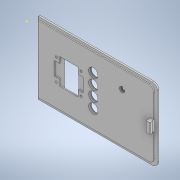
# Autodesk Inventor part: Case top
Saved by Autodesk Inventor 2021 (Build 250183000, 183)
## iProperties
Created: 2020-08-28
Part Number: Case top
Material: Generisch
Document SubType Name: Modeling
Designer: michox
Density: 1 g/cm^3
Appearance: Vorgabe
Author: michox
Autodesk Inventor part; units mm, degrees
ref_plane "YZ Plane" through (0, 0, 0) normal (1, 0, 0) x (0, 1, 0)
ref_plane "XZ Plane" through (0, 0, 0) normal (0, 1, 0) x (-1, 0, 0)
ref_plane "XY Plane" through (0, 0, 0) normal (0, 0, 1) x (1, 0, 0)
sketch "Skizze1" plane through (0, 0, 0) normal (0, 0, 1) x (1, 0, 0)
  line L0 (11.1165, 10) -> (126.7755, 10)
  line L1 (126.7755, 10) -> (126.7755, -60)
  line L2 (126.7755, -60) -> (11.1165, -60)
  line L3 (11.1165, -60) -> (11.1165, 10)
  line L4 (36.6476, -12.5) -> (50.6476, -12.5)
  line L5 (50.6476, -12.5) -> (50.6476, -37.5)
  line L6 (50.6476, -37.5) -> (36.6476, -37.5)
  line L7 (36.6476, -37.5) -> (36.6476, -12.5)
  line L8 (126.7755, -25) -> (11.1165, -25)
  line L9 (126.7755, -36.2282) -> (128.5882, -36.2282)
  line L10 (128.5882, -36.2282) -> (128.5882, -13.7718)
  line L11 (128.5882, -13.7718) -> (126.7755, -13.7718)
  line L12 (126.7755, -13.7718) -> (126.7755, -36.2282)
  circle A0 centre (65.6476, -10) radius 4.5
  circle A1 centre (65.6476, -20) radius 4.5
  circle A2 centre (65.6476, -30) radius 4.5
  circle A3 centre (65.6476, -40) radius 4.5
  circle A4 centre (93.6476, -10) radius 2.5
  point P0 (0, 0)
  dimension "d0" = 115.659
  dimension "d1" = 70
  dimension "d2" = 25
  dimension "d3" = 14
  dimension "d65" = 9
  dimension "d66" = 9
  dimension "d67" = 9
  dimension "d68" = 9
  dimension "d69" = 10
  dimension "d70" = 10
  dimension "d71" = 10
  dimension "d73" = 10
  dimension "d74" = 15
  dimension "d75" = 25.5312
  dimension "d76" = 22.5
  dimension "d77" = 5
  dimension "d79" = 28
  constraints: 26 end point, 6 parallel, 5 centre point, 3 horizontal, 3 perpendicular, 2 midpoint, 1 horizontal alignment, 1 point on line, 1 vertical alignment, 2 other
  measures "d0" distance of L1.end L2.end
  measures "d1" distance of L0.end L1.end
  measures "d2" distance of L4.end L5.end
  measures "d3" distance of L4.start L4.end
  measures "d65" diameter of A0
  measures "d66" diameter of A1
  measures "d67" diameter of A2
  measures "d68" diameter of A3
  measures "d69" distance of A1.centre A0.centre
  measures "d70" distance of A2.centre A1.centre
  measures "d71" distance of A2.centre A3.centre
  measures "d73" diameter of A1.centre L8
  measures "d74" distance from line of A2.centre L5
  measures "d75" distance between parallel lines of L3 L7
  measures "d76" distance between parallel lines of L4 L0
  measures "d77" diameter of A4
  measures "d79" distance of A4.centre A0.centre
extrude "Extrusion1" add sketch "Skizze1" along normal blind 1.5 contours L0 L1 L8 L5 L4 L7 L3 | L8 L7 L6 L5 L1 L2 L3
sketch "Skizze2" plane through (0, 0, 1.5) normal (0, 0, 1) x (1, 0, 0)
  point P0 (0, 0)
sketch "Skizze3" plane through (0, 0, 1.5) normal (0, 0, 1) x (1, 0, 0)
  line L0 (126.7755, -60) -> (126.7755, 10)
  line L1 (124.2755, -30) -> (121.2755, -30)
  line L2 (121.2755, -30) -> (121.2755, -20)
  line L3 (121.2755, -20) -> (124.2755, -20)
  line L4 (124.2755, -20) -> (124.2755, -30)
  line L5 (126.7755, -25) -> (117.2329, -25)
  line L6 (135, -36) -> (135, -24)
  line L7 (11.1165, -60) -> (126.7755, -60) projected
  line L8 (126.7755, 10) -> (11.1165, 10) projected
  point P0 (0, 0)
  dimension "d6" = 10
  dimension "d62" = 2.5
  dimension "d63" = 3
  constraints: 15 end point, 2 horizontal, 2 parallel, 2 perpendicular, 1 midpoint, 1 vertical, 1 other
  measures "d6" distance of L1.end L2.end
  measures "d62" distance between parallel lines of L4 L0
  measures "d63" distance between parallel lines of L2 L4
extrude "Extrusion2" add sketch "Skizze3" along normal blind 5.5
sketch "Skizze4" plane through (124.2755, -54, 0) normal (1, 0, 0) x (0, 0, -1)
  line L0 (-7, 24) -> (-7, 36) projected
  line L1 (-1.5, 34) -> (-7, 34) projected
  line L2 (-7, 24) -> (-4, 24)
  line L3 (-4, 24) -> (-4, 34)
  line L4 (-4, 34) -> (-7, 34)
  line L5 (-7, 34) -> (-7, 24)
  line L6 (-1.5, -6) -> (-1.5, 64) projected
  point P0 (0, 54)
  point P1 (-1.5, 24)
  point P2 (-7, 34)
  dimension "d9" = 2.5
  constraints: 8 end point, 2 parallel, 1 horizontal, 1 perpendicular, 2 other
  measures "d9" distance between parallel lines of L3 L6
extrude "Extrusion3" add sketch "Skizze4" along normal blind 0.8
chamfer "Fase1" distance 0.75 angle 45 2 edges at (125.0755, -25, 7) (125.0755, -25, 4)
chamfer "Fase2" distance 1.5 angle 45 4 edges at (36.6476, -25, 0) (43.6476, -12.5, 0) (50.6476, -25, 0) (43.6476, -37.5, 0)
chamfer "Fase3" distance 1.5 angle 30 1 edges at (11.1165, -25, 0) measured on face at (11.1165, -25, 0.5)
sketch "Skizze5" plane through (0, 0, 1.5) normal (0, 0, 1) x (1, 0, 0)
  line L0 (11.9825, 10) -> (11.9825, -60)
  line L1 (11.9825, 7.5) -> (124.2755, 7.5)
  line L2 (124.2755, 7.5) -> (124.2755, -57.5)
  line L3 (124.2755, -57.5) -> (11.9825, -57.5)
  line L4 (11.9825, -57.5) -> (11.9825, 7.5)
  line L5 (126.7755, -60) -> (126.7755, 10) projected
  line L6 (126.7755, 10) -> (11.1165, 10) projected
  line L7 (11.1165, 10) -> (11.1165, -60) projected
  line L8 (11.1165, -60) -> (126.7755, -60) projected
  line L9 (27.8476, -18.5) -> (55.8476, -18.5)
  line L10 (55.8476, -18.5) -> (55.8476, -31.5)
  line L11 (55.8476, -31.5) -> (27.8476, -31.5)
  line L12 (27.8476, -31.5) -> (27.8476, -18.5)
  line L13 (36.6476, -37.5) -> (36.6476, -12.5) projected
  line L14 (36.6476, -12.5) -> (50.6476, -12.5) projected
  line L15 (58.8722, -25) -> (36.6476, -25)
  line L16 (36.6476, -37.5) -> (50.6476, -37.5)
  line L17 (32.8476, -37.5) -> (50.8476, -37.5)
  line L18 (50.8476, -37.5) -> (50.8476, -12.5)
  line L19 (50.8476, -12.5) -> (32.8476, -12.5)
  line L20 (32.8476, -12.5) -> (32.8476, -37.5)
  line L21 (50.6476, -37.5) -> (36.6476, -37.5) projected
  line L22 (50.6476, -12.5) -> (50.6476, -37.5) projected
  circle A0 centre (93.6476, -10) radius 2.5 projected
  circle A1 centre (65.6476, -10) radius 4.5 projected
  circle A2 centre (65.6476, -20) radius 4.5 projected
  circle A3 centre (65.6476, -30) radius 4.5 projected
  circle A4 centre (65.6476, -40) radius 4.5 projected
  point P0 (0, 0)
  point P1 (135, -24)
  point P2 (36.6476, -18.5)
  point P3 (36.6476, -31.5)
  point P4 (50.8476, -31.5)
  point P5 (50.6476, -37.5)
  point P6 (36.6476, -37.5)
  point P7 (32.8476, -31.5)
  point P8 (32.8476, -18.5)
  point P9 (36.6476, -12.5)
  point P10 (50.6476, -12.5)
  point P11 (50.8476, -18.5)
  point P12 (126.7755, -13.7718)
  dimension "d21" = 2.5
  dimension "d22" = 2.5
  dimension "d24" = 2.5
  dimension "d25" = 0.866
  dimension "d26" = 28
  dimension "d27" = 13
  dimension "d28" = 8.8
  dimension "d60" = 5
  dimension "d61" = 5
  dimension "d64" = 5.2
  constraints: 30 end point, 6 parallel, 4 horizontal, 3 perpendicular, 2 collinear, 1 midpoint, 1 point on line, 3 other
  measures "d22" distance between parallel lines of L6 L1
  measures "d24" distance between parallel lines of L8 L3
  measures "d25" distance between parallel lines of L7 L0
  measures "d26" distance of L9.start L9.end
  measures "d27" distance of L9.end L10.end
  measures "d28" distance between parallel lines of L12 L13
  measures "d60" distance between parallel lines of L18 L10
  measures "d61" distance between parallel lines of L20 L12
extrude "Extrusion5" add sketch "Skizze5" along normal blind 1 contours L1 L2 L3 L0
sketch "Skizze6" plane through (0, 0, 2.5) normal (0, 0, 1) x (1, 0, 0)
  line L0 (27.8476, -31.5) -> (27.8476, -18.5) projected
  line L1 (55.8476, -18.5) -> (55.8476, -31.5) projected
  line L2 (36.6476, -12.5) -> (50.6476, -12.5) projected
  line L3 (50.6476, -37.5) -> (36.6476, -37.5) projected
  point P0 (0, 0)
  point P1 (29.8476, -35.5)
  point P2 (29.8476, -14.5)
  point P3 (53.8476, -35.5)
  point P4 (53.8476, -14.5)
  dimension "d36" = 2
  dimension "d37" = 2
  dimension "d38" = 2
  dimension "d39" = 2
  dimension "d40" = 2
  dimension "d41" = 2
  dimension "d42" = 2
  constraints: 1 horizontal alignment
  measures "d36" distance from line of point (29.848, -35.5) L0
  measures "d37" distance from line of point (29.848, -14.5) L0
  measures "d38" distance from line of L1 point (53.848, -35.5)
  measures "d39" distance from line of L1 point (53.848, -14.5)
  measures "d40" distance from line of point (53.848, -14.5) L2
  measures "d41" distance from line of point (53.848, -35.5) L3
  measures "d42" distance from line of L3 point (29.848, -35.5)
hole "Bohrung1" at (29.8476, -35.5, 2.5) at (29.8476, -14.5, 2.5) at (53.8476, -35.5, 2.5) at (53.8476, -14.5, 2.5) direction (0, 0, -1) diameter 2 depth 2.25
fillet "Rundung1" radius 4.75 4 edges at (126.7755, 10, 0.75) (126.7755, -60, 0.75) (124.2755, -57.5, 2) (124.2755, 7.5, 2)
